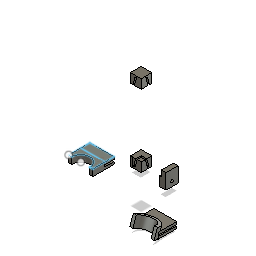
Plexiglass Holders (Autodesk Fusion 360 design; units mm, degrees)
Autodesk Fusion 360 part; units mm, degrees
note: some values were not read from the file. Set by a fixed rule: which sketch regions a step uses.
sketch "Sketch1" plane through (0, 0, 0) normal (0, 1, 0) x (1, 0, 0)
  line L0 (0, 0) -> (406.4, 0)
  line L1 (406.4, 0) -> (406.4, -279.4)
  line L2 (406.4, -279.4) -> (0, -279.4)
  line L3 (0, -279.4) -> (0, 0)
  line L4 (404.0378, -277.0378) -> (2.3622, -277.0378)
  line L5 (2.3622, -277.0378) -> (2.3622, -2.3622)
  line L6 (2.3622, -2.3622) -> (404.0378, -2.3622)
  line L7 (404.0378, -2.3622) -> (404.0378, -277.0378)
  dimension "d1" = 406.4
  dimension "d2" = 279.4
  dimension "d7" = 2.3622
  constraint horizontal L0
  constraint vertical L1
  constraint horizontal L2
  constraint vertical L3
  constraint coincident L0.start L3.end
  measures "d1" distance of L0.start L0.end
  measures "d2" distance of L0.start L2.end
ref_plane "WorkPlane1" through (203.2, 177.8, 139.7) normal (0, 1, 0) x (1, 0, 0)
sketch "Sketch2" plane through (203.2, 177.8, 139.7) normal (0, 1, 0) x (1, 0, 0)
  line L0 (152.4, -88.9) -> (-152.4, -88.9)
  line L1 (-152.4, -88.9) -> (-152.4, 88.9)
  line L2 (-152.4, 88.9) -> (152.4, 88.9)
  line L3 (152.4, 88.9) -> (152.4, -88.9)
  line L4 (150.0378, -86.5378) -> (-150.0378, -86.5378)
  line L5 (-150.0378, -86.5378) -> (-150.0378, 86.5378)
  line L6 (-150.0378, 86.5378) -> (150.0378, 86.5378)
  line L7 (150.0378, 86.5378) -> (150.0378, -86.5378)
  dimension "d8" = 2.3622
loft "Loft1" add profiles "Sketch1", "Sketch2" section 1 contours L0 L1 L2 L3 | L4 L5 L6 L7 section 2 contours L0 L1 L2 L3 | L4 L5 L6 L7 makes body 1 in component "Component"
loft "Loft3" cut profiles "Sketch1", "Sketch2" section 1 contours L4 L5 L6 L7 section 2 contours L4 L5 L6 L7 bodies 1 in component "Component"
sketch "Sketch3" plane through (0, 0, 0) normal (0, 1, 0) x (1, 0, 0)
  line L0 (12.7, -12.7) -> (-1.27, -12.7)
  line L1 (12.7, 1.27) -> (12.7, -12.7)
  line L2 (12.7, -12.7) -> (-12.7, 12.7) construction
  line L3 (-12.7, -12.7) -> (12.7, 12.7) construction
  line L4 (12.7, 1.27) -> (12.7, -12.7)
  line L5 (12.7, -12.7) -> (-1.27, -12.7)
  line L6 (12.7, 1.27) -> (12.7, 5.08)
  line L7 (12.7, 5.08) -> (-5.08, 5.08)
  line L8 (-5.08, -12.7) -> (-1.27, -12.7)
  line L9 (-5.08, -12.7) -> (-5.08, 5.08)
  dimension "d9" = 25.4
  dimension "d10" = 25.4
  constraint horizontal L0
  constraint coincident L2 origin
  constraint coincident L3 origin
  constraint coincident L2 L7.end
  constraint perpendicular L6 L7
  constraint perpendicular L7 L9
  measures "d9" distance of L3.start L2.end
  measures "d10" horizontal distance of L2.end L3.end
extrude "Extrude1" add sketch "Sketch3" along normal blind 12.7 separate body makes body 2
extrude "Extrude3" add sketch "Sketch3" against normal blind 2.54 bodies 2
combine "Combine1" operation cut target body 2 tool bodies 1 keep tools
sketch "Sketch4" plane through (203.2, 177.8, 139.7) normal (0, 1, 0) x (1, 0, 0)
  line L0 (-139.7, 76.2) -> (-153.67, 76.2)
  line L1 (-139.7, 90.17) -> (-139.7, 76.2)
  line L2 (-139.7, 76.2) -> (-165.1, 101.6) construction
  line L3 (-165.1, 76.2) -> (-139.7, 101.6) construction
  line L4 (-139.7, 76.2) -> (-139.7, 90.17)
  line L5 (-153.67, 90.17) -> (-153.67, 90.17)
  line L6 (-153.67, 76.2) -> (-139.7, 76.2)
  line L7 (-139.7, 90.17) -> (-139.7, 93.98)
  line L8 (-139.7, 93.98) -> (-157.48, 93.98)
  line L9 (-153.67, 76.2) -> (-157.48, 76.2)
  line L10 (-157.48, 76.2) -> (-157.48, 93.98)
  point P0 (-152.4, 88.9)
  point P1 (-152.4, 88.9)
  dimension "d17" = 25.4
  dimension "d18" = 25.4
  constraint horizontal L0
  constraint coincident L2 P1
  constraint coincident L3 P1
  constraint coincident P1 P0
  constraint parallel L4 L5
  constraint coincident L2 L8.end
  constraint perpendicular L7 L8
  constraint perpendicular L5 L9
  constraint perpendicular L8 L10
  measures "d17" distance of L2.end L3.end
  measures "d18" distance of L3.start L2.end
extrude "Extrude4" add sketch "Sketch4" along normal blind 2.54 separate body makes body 3
extrude "Extrude5" add 1 faces at (52.9167, 177.8, 52.9167) along direction (0, -1, 0) blind 12.7 on bodies 3 bodies 3
move_body "Move1" bodies 3 to x (1, 0, 0) y (0, 1, 0) z (0, 0, 1) at (-2.54, 0, -2.54)
combine "Combine2" operation cut target body 3 tool bodies 1 keep tools
sketch "Sketch5" plane through (0, 0, 0) normal (0, 1, 0) x (1, 0, 0)
  line L0 (50, 0) -> (61, 0)
  line L1 (61, 0) -> (61, -20)
  line L2 (61, -20) -> (50, -20)
  line L3 (50, -20) -> (50, 0)
  line L4 (50, 0) -> (53.175, 0)
  line L5 (53.175, 0) -> (53.175, -20)
  line L6 (53.175, -20) -> (50, -20)
  line L7 (50, -20) -> (50, 0)
  dimension "d26" = 3.175
  dimension "d45" = 11
  constraint perpendicular L0 L1
  constraint parallel L0 L2
  constraint parallel L1 L3
  constraint horizontal L0
  constraint perpendicular L4 L5
  constraint parallel L4 L6
  constraint parallel L5 L7
  constraint perpendicular L3 L4
  measures "d26" distance of L0.start L4.end
  measures "d45" horizontal distance of L0.start L0.end
extrude "Extrude6" add sketch "Sketch5" along normal blind 25 separate body contours L0 L1 L2 L5 makes body 4
extrude "Extrude8" add sketch "Sketch5" along normal blind 15 contours L0 L2 L3 L4 L5 L6 L7 bodies 4
sketch "Sketch8" plane through (61, 0, 0) normal (1, 0, 0) x (0, 0, -1)
  line L0 (-20, 0) -> (0, 0)
  line L1 (0, 0) -> (0, 25)
  line L2 (0, 25) -> (-20, 25)
  line L3 (-20, 25) -> (-20, 0)
  circle A0 centre (-10, 8) radius 2.25
  circle A1 centre (-10, 8) radius 1.8
  dimension "d39" = 4.5
  dimension "d40" = 3.6
  constraint concentric A0 A1
  measures "d39" diameter of A0
  measures "d40" diameter of A1
extrude "Extrude10" cut sketch "Sketch8" against normal up to surface (11 mm away) contours A1 bodies 4
extrude "Extrude11" cut sketch "Sketch8" against normal blind 3.6 contours A0 bodies 4
sketch "Sketch9" plane through (0, 0, 0) normal (0, 1, 0) x (1, 0, 0)
  arc A0 (115, -100) -> (85, -100) centre (100, -100) ccw
  arc A1 (120, -100) -> (80, -100) centre (100, -100) ccw
  line L0 (120, -100) -> (115, -100)
  line L1 (85, -100) -> (80, -100)
  line L2 (120, -100) -> (120, -60)
  line L3 (120, -60) -> (80, -60)
  line L4 (80, -60) -> (80, -100)
  line L5 (80, -90.037) -> (82.6582, -90.037)
  line L6 (117.3418, -90.037) -> (120, -90.037)
  dimension "d47" = 40
  constraint horizontal L0
  constraint coincident A0.end L0
  constraint collinear L0 L1
  constraint tangent A1 L2
  constraint perpendicular L0 L2
  constraint perpendicular L2 L3
  constraint tangent A1 L4
  constraint coincident L4 L5.start
  constraint coincident L2 L6.end
  constraint perpendicular L2 L5
  constraint coincident A1 L6.start
  constraint collinear L5 L6
  constraint coincident A1 L5.end
  measures "d47" distance of A0.centre L3
extrude "Extrude17" add sketch "Sketch9" along normal blind 17 separate body contours A0 A1 L0 L1 makes body 5
move_body "Move3" bodies 5 to x (1, 0, 0) y (0, 0.939693, -0.34202) z (0, 0.34202, 0.939693) at (0, -27.3616, 4.8246)
move_body "Move4" bodies 5 to x (1, 0, 0) y (0, 1, 0) z (0, 0, 1) at (0, -3, 0)
extrude "Extrude18" add sketch "Sketch9" along normal blind 4 contours A1 L2 L3 L4 L5 L6 bodies 5
move_body "Move5" bodies 5 to x (1, 0, 0) y (0, 1, 0) z (0, 0, 1) at (0, -7, 0)
extrude "Extrude19" add sketch "Sketch9" along normal blind 4 contours A1 L2 L3 L4 L5 L6 bodies 5
extrude "Extrude20" cut 1 faces at (120, 1.3333, 80.0246) along direction (-1, 0, 0) blind 1 on bodies 5 bodies 5
extrude "Extrude21" cut 1 faces at (80, 2.6667, 70.0123) along direction (1, 0, 0) blind 1 on bodies 5 bodies 5
extrude "Extrude22" cut 1 faces at (80, -4.3333, 70.0123) along direction (1, 0, 0) blind 2 on bodies 5 bodies 5
extrude "Extrude23" cut 1 faces at (120, -5.6667, 80.0246) along direction (-1, 0, 0) blind 2 on bodies 5 bodies 5
sketch "Sketch11" plane through (0, 0, 0) normal (0, 1, 0) x (1, 0, 0)
  arc A0 (-35, -50) -> (-65, -50) centre (-50, -50) ccw
  line L0 (-70, -50) -> (-65, -50)
  line L1 (-35, -50) -> (-30, -50)
  line L2 (-30, -50) -> (-30, -15)
  line L3 (-30, -15) -> (-70, -15)
  line L4 (-70, -15) -> (-70, -50)
  line L5 (-70, -30) -> (-30, -30)
  line L6 (-70, -50) -> (-65, -50)
  line L7 (-35, -50) -> (-30, -50)
  dimension "d73" = 30
  dimension "d75" = 35
  constraint horizontal L0
  constraint coincident A0.start L0
  constraint collinear L0 L1
  constraint perpendicular L2 L3
  constraint parallel L2 L4
  constraint parallel L3 L6
  constraint perpendicular L1 L2
  constraint coincident L4 L5.start
  constraint coincident L2 L5.end
  constraint perpendicular L2 L5
  constraint collinear L6 L7
  measures "d73" diameter of A0
  measures "d75" vertical distance of L1.end L2.end
extrude "Extrude24" add sketch "Sketch11" along normal blind 4 separate body makes body 6
extrude "Extrude25" add sketch "Sketch11" along normal blind 11 contours A0 L0 L1 L2 L4 L5 L6 L7 bodies 6
move_body "Move6" bodies 6 to x (1, 0, 0) y (0, 1, 0) z (0, 0, 1) at (0, -11, 0)
extrude "Extrude26" add sketch "Sketch11" against normal blind 4 contours L2 L3 L4 L5 bodies 6
component "Component" placed x (1, 0, 0) y (0, 1, 0) z (0, 0, 1) at (0, 0, 0)
hidden bodies 1
named bodies: "Cover", "Bottom Plexi", "Top Plexi", "Plexi Holder", "Angled Holder", "Straight Holder"
